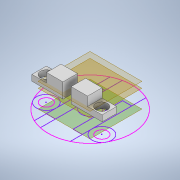
# Autodesk Inventor part: cover
Saved by Autodesk Inventor 2020 (Build 240168000, 168)
## iProperties
Created: 2019-06-14
Part Number: cover
Material: Generic
Document SubType Name: Modeling
Designer: ColinP
Density: 1 g/cm^3
Appearance: Default
Mass: 11.1656 g
Surface Area: 41.7742 cm^2
Volume: 11.1656 cm^3
Author: ColinP
Autodesk Inventor part; units mm, degrees
ref_plane "YZ Plane" through (0, 0, 0) normal (1, 0, 0) x (0, 1, 0)
ref_plane "XZ Plane" through (0, 0, 0) normal (0, 1, 0) x (-1, 0, 0)
ref_plane "XY Plane" through (0, 0, 0) normal (0, 0, 1) x (1, 0, 0)
ref_plane "Work Plane1" through (0, 0, 0) normal (0, -1, 0) x (1, 0, 0)
sketch "Sketch14" plane through (0, 0, 0) normal (0, -1, 0) x (1, 0, 0)
  circle A0 centre (11.7904, 6.8072) radius 2.4511 projected
  circle A1 centre (0, -13.6144) radius 2.4511 projected
  circle A2 centre (-11.7904, 6.8072) radius 2.4511 projected
  point P0 (0, 0)
ref_plane "Work Plane3" through (0, 0, 0) normal (0, -1, 0) x (1, 0, 0)
sketch "Sketch18" plane through (0, 0, 0) normal (0, -1, 0) x (1, 0, 0)
  circle A0 centre (-11.7904, 6.8072) radius 2.4511 projected
  circle A1 centre (-11.7904, 6.8072) radius 4.1697
  circle A2 centre (0, 0) radius 3.7517
  line L0 (-7.6207, 6.8072) -> (-7.6207, -16.064)
  circle A3 centre (0, 0) radius 17.78 projected
  line L1 (-7.6207, 6.8072) -> (-7.6207, 16.064)
  line L2 (-3.7517, 0) -> (-3.7517, -17.4687)
  line L3 (-3.7517, -17.4687) -> (-3.7517, 17.2429)
  circle A4 centre (11.7904, 6.8072) radius 2.4511 projected
  circle A5 centre (11.7904, 6.8072) radius 4.1697
  line L4 (7.6207, 6.8072) -> (7.6207, -16.064)
  line L5 (7.6207, 16.064) -> (7.6207, 6.8072)
  line L6 (-7.6207, 10.9769) -> (-3.7517, 10.9769)
  line L7 (-6.9141, -9.9949) -> (-3.7517, -9.9949)
  line L8 (-7.6207, -9.9949) -> (-6.5754, -9.9949)
  line L9 (3.7517, 10.9769) -> (7.6207, 10.9769)
  line L10 (3.7517, -9.9949) -> (7.6207, -9.9949)
  line L11 (0, 0) -> (3.7517, 0)
  line L12 (3.7517, 0) -> (3.7517, 10.8227)
  line L13 (3.7517, 10.8227) -> (3.7517, -9.9949)
  line L14 (3.7517, 10.8227) -> (3.7517, 10.9769)
  line L15 (7.6207, 10.9769) -> (3.7517, 10.9769)
  point P0 (3.7517, 0)
  constraints: 32 end point, 15 point on line, 6 point on circle, 4 vertical, 3 coincident, 3 collinear, 2 horizontal alignment, 2 perpendicular, 1 centre point, 1 horizontal, 1 parallel, 1 tangent, 4 other
ref_plane "Work Plane4" through (0, 7.62, 0) normal (0, 1, 0) x (1, 0, 0)
sketch "Sketch19" plane through (0, 7.62, 0) normal (0, 1, 0) x (1, 0, 0)
  circle A0 centre (0, 0) radius 17.78 projected
  line L0 (1.7319, -3.6013) -> (14.874, -3.6013)
  line L1 (14.874, -3.6013) -> (14.874, -9.7412)
  line L2 (14.874, -9.7412) -> (1.7319, -9.7412)
  line L3 (1.7319, -9.7412) -> (1.7319, -3.6013)
  constraints: 8 end point, 2 parallel, 1 horizontal, 1 perpendicular, 2 other
extrude "Extrusion7" add sketch "Sketch19" along normal blind 2.54 contours L2 L3 L0 L1
ref_plane "Work Plane5" through (0, 10.16, 0) normal (0, 1, 0) x (1, 0, 0)
sketch "Sketch20" plane through (0, 10.16, 0) normal (0, 1, 0) x (1, 0, 0)
  circle A0 centre (11.7904, -6.8072) radius 2.4511 projected
  circle A1 centre (11.7904, -6.8072) radius 2.4511
  line L0 (7.6207, -3.6013) -> (14.874, -3.6013) projected
  line L1 (8.7038, -3.6013) -> (8.7038, -9.7412)
  line L2 (3.7517, -9.7412) -> (1.7319, -9.7412) projected
  line L3 (8.7038, -9.7412) -> (1.7319, -9.7412)
  line L4 (1.7319, -9.7412) -> (1.7319, -3.6013) projected
  line L5 (1.7319, -9.7412) -> (1.7319, -3.6013)
  line L6 (1.7319, -3.6013) -> (8.7038, -3.6013)
  point P0 (0, 0)
  constraints: 8 end point, 2 collinear, 1 centre point, 1 coincident, 1 perpendicular, 1 point on line, 1 vertical
extrude "Extrusion8" add sketch "Sketch20" along normal blind 3.81 contours L0 L1 L3 L2 L4 L6
hole "Hole5" at (11.7904, 0, 6.8072) direction (0, 1, 0) diameter 4.9022 end through all
ref_plane "Work Plane2" through (0, 7.62, 0) normal (0, 1, 0) x (1, 0, 0)
sketch "Sketch21" plane through (0, 7.62, 0) normal (0, 1, 0) x (1, 0, 0)
  circle A0 centre (-11.7904, -6.8072) radius 2.4511 projected
  line L0 (-14.239, -6.6967) -> (-14.874, -6.6967)
  line L1 (1.7319, -9.7412) -> (1.7319, -3.6013) projected
  line L2 (1.7319, -3.6013) -> (-14.874, -3.6013)
  line L3 (-14.874, -3.6013) -> (-14.874, -6.6967)
  line L4 (1.7319, -9.7412) -> (-14.874, -9.7412)
  circle A1 centre (0, 0) radius 17.78 projected
  line L5 (-14.874, -6.6967) -> (-14.874, -9.7412)
  line L6 (-3.7517, 9.9949) -> (-3.7517, -10.9769) projected
  line L7 (-3.7517, -3.6013) -> (-1.7197, -3.6013)
  line L8 (-1.7197, -3.6013) -> (-1.7197, -9.7412)
  line L9 (-14.874, -9.7412) -> (-14.874, -3.6013)
  dimension "d67" = 0.635
  dimension "d68" = 2.032
  constraints: 16 end point, 4 point on line, 3 horizontal, 3 perpendicular, 1 collinear, 4 other
  measures "d67" distance of L0.start L0.end
  measures "d68" distance of L7.start L7.end
extrude "Extrusion9" add sketch "Sketch21" along normal blind 2.54 contours L4 L6 L2 L8 | L4 L5 L3 L2 L6
sketch "Sketch22" plane through (0, 10.16, 0) normal (0, 1, 0) x (1, 0, 0)
  point P0 (0, 0)
sketch "Sketch23" plane through (0, 10.16, 0) normal (0, 1, 0) x (1, 0, 0)
  line L0 (8.7038, -3.6013) -> (1.7319, -3.6013) projected
  line L1 (-1.7197, -9.7412) -> (-1.7197, -3.6013) projected
  line L2 (-1.7197, -3.6013) -> (-8.6793, -3.6013)
  line L3 (-1.7197, -3.6013) -> (-14.874, -3.6013) projected
  line L4 (-8.6793, -3.6013) -> (-8.6793, -9.7412)
  line L5 (-14.874, -9.7412) -> (-1.7197, -9.7412) projected
  line L6 (-8.6793, -9.7412) -> (-1.7197, -9.7412)
  line L7 (-1.7197, -9.7412) -> (-1.7197, -3.6013)
  point P0 (0, 0)
  dimension "d71" = 6.9596
  constraints: 8 end point, 3 perpendicular, 1 point on line
  measures "d71" distance of L1.end L2.end
extrude "Extrusion10" add sketch "Sketch23" along normal blind 3.81
body "Solid1"
